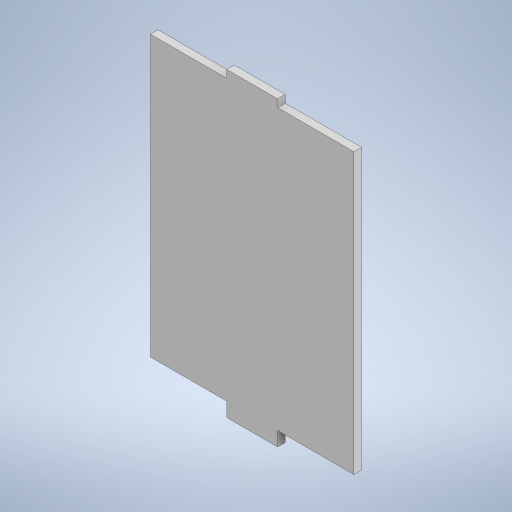
# Autodesk Inventor part: SideWallV2
Saved by Autodesk Inventor 2023 (Build 270158000, 158)
## iProperties
Created: 2022-10-06
Part Number: SideWallV2
Material: Generic
Document SubType Name: Modeling
Designer: digge
Density: 1 g/cm^3
Appearance: Default
Author: digge
Autodesk Inventor part; units mm, degrees
ref_plane "YZ Plane" through (0, 0, 0) normal (1, 0, 0) x (0, 1, 0)
ref_plane "XZ Plane" through (0, 0, 0) normal (0, 1, 0) x (-1, 0, 0)
ref_plane "XY Plane" through (0, 0, 0) normal (0, 0, 1) x (1, 0, 0)
sketch "Sketch1" plane through (0, 0, 0) normal (0, 0, 1) x (1, 0, 0)
  line L0 (-88.1992, 54.8893) -> (-88.1992, -55.1107)
  line L1 (-88.1992, -55.1107) -> (-58.1992, -55.1107)
  line L2 (-58.1992, -55.1107) -> (-58.1992, -60.7107)
  line L3 (-58.1992, -60.7107) -> (-38.1992, -60.7107)
  line L4 (-38.1992, -60.7107) -> (-38.1992, -55.1107)
  line L5 (-38.1992, -55.1107) -> (-8.1992, -55.1107)
  line L6 (-8.1992, -55.1107) -> (-8.1992, 54.8893)
  line L7 (-8.1992, 54.8893) -> (-38.1992, 54.8893)
  line L8 (-38.1992, 54.8893) -> (-38.1992, 57.8893)
  line L9 (-38.1992, 57.8893) -> (-58.1992, 57.8893)
  line L10 (-58.1992, 57.8893) -> (-58.1992, 54.8893)
  line L11 (-88.1992, 54.8893) -> (-58.1992, 54.8893)
  point P0 (0, 0)
  dimension "d0" = 110
  dimension "d1" = 20
  dimension "d2" = 80
  dimension "d3" = 30
  dimension "d6" = 3
  dimension "d7" = 5.6
  constraints: 24 end point, 7 perpendicular, 7 point on line, 1 horizontal, 1 vertical
  measures "d0" distance of L0.start L0.end
  measures "d1" distance of L8.end L9.end
  measures "d2" distance between parallel lines of L6 L0
  measures "d3" distance of L6.end L7.end
  measures "d6" distance of L7.end L8.end
  measures "d7" distance between parallel lines of L5 L3
extrude "Extrusion1" add sketch "Sketch1" along normal blind 3
body "Solid1"
